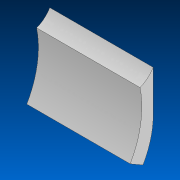
# Autodesk Inventor part: FlyWheel Alligner
Saved by Autodesk Inventor 2022 (Build 260153000, 153)
## iProperties
Created: 2022-04-25
Part Number: FlyWheel Alligner
Material: Generic
Document SubType Name: Modeling
Designer: score_nygvs6w
Density: 1 g/cm^3
Appearance: Default
Author: score_nygvs6w
Autodesk Inventor part; units mm, degrees
ref_plane "YZ Plane" through (0, 0, 0) normal (1, 0, 0) x (0, 1, 0)
ref_plane "XZ Plane" through (0, 0, 0) normal (0, 1, 0) x (-1, 0, 0)
ref_plane "XY Plane" through (0, 0, 0) normal (0, 0, 1) x (1, 0, 0)
sketch "Sketch1" plane through (0, 0, 0) normal (1, 0, 0) x (0, 1, 0)
  line L0 (-219.6367, 33.4515) -> (-197.6397, 20.7515)
  line L1 (-197.6397, 20.7515) -> (-184.9397, 42.7485)
  line L2 (-184.9397, 42.7485) -> (-206.9367, 55.4485)
  line L3 (-206.9367, 55.4485) -> (-219.6367, 33.4515)
  line L4 (-219.6367, 33.4515) -> (-184.9397, 42.7485) construction
  line L5 (-197.6397, 20.7515) -> (-206.9367, 55.4485) construction
  circle A0 centre (-38.1, 41.275) radius 38.1
  line L6 (0, 0) -> (-228.6, 0)
  line L7 (-228.6, 0) -> (-228.6, -25.4)
  line L8 (-228.6, -25.4) -> (0, -25.4)
  line L9 (0, -25.4) -> (0, 0)
  line L10 (0, 0) -> (-228.6, -25.4) construction
  line L11 (-228.6, 0) -> (0, -25.4) construction
  line L12 (-38.1, 3.175) -> (-132.0434, 3.175)
  arc A1 (-197.6397, 20.7515) -> (-132.0434, 3.175) centre (-132.0434, 134.3676) ccw
  circle A2 centre (-38.1, 41.275) radius 44.45
  arc A3 (-184.9397, 42.7485) -> (-79.7897, 25.8552) centre (-110.2136, 172.1778) ccw
  circle A4 centre (-101.6, 41.275) radius 7.3323
  line L13 (-107.95, 44.9412) -> (-101.6, 48.6073)
  line L14 (-101.6, 48.6073) -> (-95.25, 44.9412)
  line L15 (-95.25, 44.9412) -> (-95.25, 37.6088)
  line L16 (-95.25, 37.6088) -> (-101.6, 33.9427)
  line L17 (-101.6, 33.9427) -> (-107.95, 37.6088)
  line L18 (-107.95, 37.6088) -> (-107.95, 44.9412)
  point P0 (-202.2882, 38.1)
  point P1 (-114.3, -12.7)
  point P2 (-60.9953, 3.175)
  dimension "d0" = 76.2
  dimension "d1" = 25.4
  dimension "d2" = 60
  dimension "d3" = 41.275
  dimension "d4" = 38.1
  dimension "d5" = 146.847
  dimension "d6" = 20.7515
  dimension "d7" = 228.6
  dimension "d8" = 88.9
  dimension "d23" = 12.7
  dimension "d24" = 63.5
  constraints: 38 end point, 7 point on circle, 4 midpoint, 4 parallel, 3 centre point, 3 horizontal, 3 point on line, 3 tangent, 2 coincident, 2 equal length, 2 perpendicular, 1 horizontal alignment, 1 vertical, 1 vertical alignment, 18 other
  measures "d1" distance of L0.end L1.end
  measures "d2" angle of L1 L6
  measures "d3" distance from line of point (-38.1, 41.275) L6
  measures "d4" distance from line of L9 point (-38.1, 41.275)
  measures "d5" distance of point (-38.1, 41.275) L1.end
  measures "d6" distance from line of L6 L0.end
  measures "d7" distance of L7.end L8.end
  measures "d8" diameter of A2
  measures "d23" distance between parallel lines of L17 L14
  measures "d24" distance of point (-38.1, 41.275) point (-101.6, 41.275)
extrude "Extrusion1" add sketch "Sketch1" along normal mid plane 177.8 contours L1 A3 A2 L12 A1
sketch "Sketch2" plane through (-88.9, -197.6397, 20.7515) normal (0, -0.866, 0.5) x (1, 0, 0)
  line L0 (0, 0) -> (177.8, 0) projected
  line L1 (177.8, 25.4) -> (177.8, 0) projected
  point P0 (88.9, 80.8485)
  point P1 (152.4, 12.7)
  dimension "d11" = 12.7
  dimension "d12" = 25.4
  measures "d11" distance from line of L0 point (152.4, 12.7)
  measures "d12" distance from line of point (152.4, 12.7) L1
hole "Hole1" at (63.5, -191.2897, 31.75) direction (0, 0.866, -0.5) diameter 4.445 depth 38.1 counterbore diameter 5.588 counterbore depth 8.255
pattern_linear "Rectangular Pattern1" count 6 spacing 25.4 along (-1, 0, 0) of "Hole1"
body "Solid1"
